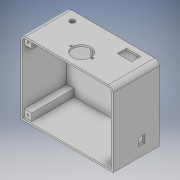
# Autodesk Inventor part: main_with_lid
Saved by Autodesk Inventor 2019 (Build 230136000, 136)
## iProperties
Created: 2019-03-27
Part Number: main_with_lid
Material: Generic
Document SubType Name: Modeling
Designer: hayes107
Density: 1 g/cm^3
Appearance: Default
Author: hayes107
Autodesk Inventor part; units mm, degrees
ref_plane "YZ Plane" through (0, 0, 0) normal (1, 0, 0) x (0, 1, 0)
ref_plane "XZ Plane" through (0, 0, 0) normal (0, 1, 0) x (-1, 0, 0)
ref_plane "XY Plane" through (0, 0, 0) normal (0, 0, 1) x (1, 0, 0)
sketch "Sketch1" plane through (0, 0, 0) normal (0, 0, 1) x (1, 0, 0)
  line L0 (0, 132.6086) -> (127, 132.6086)
  line L1 (127, 132.6086) -> (127, 31.0086)
  line L2 (127, 31.0086) -> (0, 31.0086)
  line L3 (0, 31.0086) -> (0, 132.6086)
  point P0 (0, 0)
  dimension "d0" = 101.6
  dimension "d1" = 127
  constraints: 8 end point, 2 parallel, 1 horizontal, 1 perpendicular
  measures "d0" distance between parallel lines of L2 L0
  measures "d1" distance between parallel lines of L1 L3
extrude "Extrusion1" add sketch "Sketch1" along normal blind 63.5
fillet "Fillet1" radius 6.35 1 edges at (127, 132.6086, 31.75)
fillet "Fillet2" radius 6.35 1 edges at (0, 132.6086, 31.75)
shell "Shell1" thickness 2.54 removed faces 1 at (82.55, 64.8753, 63.5)
sketch "Sketch16" plane through (0, 0, 0) normal (0, 0, -1) x (-1, 0, 0)
  line L0 (-91.3384, 109.6724) -> (-35.6616, 109.6724)
  line L1 (-35.6616, 109.6724) -> (-35.6616, 69.1086)
  line L2 (-35.6616, 69.1086) -> (-91.3384, 69.1086)
  line L3 (-91.3384, 69.1086) -> (-91.3384, 109.6724)
  line L4 (-127, 31.0086) -> (0, 31.0086) projected
  line L5 (0, 31.0086) -> (0, 126.2586) projected
  point P0 (0, 0)
  dimension "d69" = 40.5638
  dimension "d70" = 55.6768
  dimension "d71" = 38.1
  dimension "d72" = 35.6616
  constraints: 8 end point, 2 parallel, 1 horizontal, 1 perpendicular
  measures "d69" distance between parallel lines of L2 L0
  measures "d70" distance between parallel lines of L1 L3
  measures "d71" distance between parallel lines of L4 L2
  measures "d72" distance between parallel lines of L5 L1
extrude "Extrusion5" cut sketch "Sketch16" against normal blind 2.54
sketch "Sketch17" plane through (0, 0, 0) normal (0, 0, -1) x (-1, 0, 0)
  line L0 (-91.3384, 69.1086) -> (-91.3384, 109.6724) projected
  line L1 (-91.3384, 109.6724) -> (-35.6616, 109.6724) projected
  line L2 (-35.6616, 69.1086) -> (-91.3384, 69.1086) projected
  line L3 (-35.6616, 109.6724) -> (-35.6616, 69.1086) projected
  point P0 (0, 0)
  point P1 (-94.1832, 106.8276)
  point P2 (-94.1832, 71.9534)
  point P3 (-32.8168, 71.9534)
  point P4 (-32.8168, 106.8276)
  dimension "d75" = 2.8448
  dimension "d76" = 2.8448
  dimension "d77" = 2.8448
  dimension "d78" = 2.8448
  dimension "d305" = 2.8448
  dimension "d306" = 2.8448
  dimension "d307" = 2.8448
  measures "d75" distance from line of L0 point (-94.183, 106.828)
  measures "d76" distance from line of L1 point (-94.183, 106.828)
  measures "d77" distance from line of L2 point (-94.183, 71.953)
  measures "d78" distance from line of L3 point (-32.817, 71.953)
  measures "d305" distance from line of L2 point (-32.817, 71.953)
  measures "d306" distance from line of L3 point (-32.817, 106.828)
  measures "d307" distance from line of L1 point (-32.817, 106.828)
hole "Hole2" at (32.8168, 106.8276, 0) at (32.8168, 71.9534, 0) at (94.1832, 71.9534, 0) at (94.1832, 106.8276, 0) direction (0, 0, 1) diameter 2.6416 depth 12.7 tip angle 118
sketch "Sketch18" plane through (127, 31.0086, 63.5) normal (1, 0, 0) x (0, 0, -1)
  line L0 (35.052, 24.0792) -> (43.18, 24.0792)
  line L1 (43.18, 24.0792) -> (43.18, 13.6652)
  line L2 (43.18, 13.6652) -> (35.052, 13.6652)
  line L3 (35.052, 13.6652) -> (35.052, 24.0792)
  line L4 (63.5, 95.25) -> (63.5, 0) projected
  line L5 (63.5, 0) -> (0, 0) projected
  point P0 (63.5, -31.0086)
  dimension "d86" = 20.32
  dimension "d87" = 8.128
  dimension "d88" = 10.414
  dimension "d89" = 13.6652
  constraints: 8 end point, 2 parallel, 1 horizontal, 1 perpendicular
  measures "d86" distance between parallel lines of L4 L1
  measures "d87" distance between parallel lines of L3 L1
  measures "d88" distance between parallel lines of L2 L0
  measures "d89" distance between parallel lines of L2 L5
extrude "Extrusion6" cut sketch "Sketch18" against normal blind 2.54
sketch "Sketch26" plane through (120.65, 132.6086, 63.5) normal (0, 1, 0) x (1, 0, 0)
  line L0 (-107.95, 2.54) -> (-120.65, 2.54)
  line L1 (-120.65, 2.54) -> (-120.65, 63.5)
  line L2 (-120.65, 63.5) -> (-107.95, 63.5)
  line L3 (-107.95, 63.5) -> (-107.95, 2.54)
  line L4 (-120.65, 63.5) -> (-120.65, 0) projected
  line L5 (0, 0) -> (-114.3, 0) projected
  line L6 (-114.3, 63.5) -> (0, 63.5) projected
  line L7 (6.35, 31.75) -> (-6.35, 31.75)
  line L8 (-6.35, 31.75) -> (-6.35, 2.54)
  line L9 (-6.35, 2.54) -> (6.35, 2.54)
  line L10 (6.35, 2.54) -> (6.35, 31.75)
  line L11 (6.35, 0) -> (6.35, 63.5) projected
  dimension "d111" = 0
  dimension "d112" = 2.54
  dimension "d113" = 12.7
  dimension "d117" = 0
  dimension "d118" = 12.7
  dimension "d119" = 0
  dimension "d120" = 31.75
  dimension "d121" = 2.54
  constraints: 16 end point, 4 parallel, 2 horizontal, 2 perpendicular
  measures "d111" distance between parallel lines of L4 L1
  measures "d112" distance between parallel lines of L5 L0
  measures "d113" distance between parallel lines of L3 L1
  measures "d117" distance between parallel lines of L6 L2
  measures "d118" distance between parallel lines of L8 L10
  measures "d119" distance between parallel lines of L11 L10
  measures "d120" distance between parallel lines of L6 L7
  measures "d121" distance between parallel lines of L5 L9
sketch "Sketch27" plane through (0, 31.0086, 0) normal (0, -1, 0) x (1, 0, 0)
  line L0 (114.3, 60.96) -> (127, 60.96)
  line L1 (127, 60.96) -> (127, 31.75)
  line L2 (127, 31.75) -> (114.3, 31.75)
  line L3 (114.3, 31.75) -> (114.3, 60.96)
  line L4 (0, 63.5) -> (127, 63.5) projected
  line L5 (127, 0) -> (127, 63.5) projected
  line L6 (127, 0) -> (0, 0) projected
  line L7 (0, 60.96) -> (12.7, 60.96)
  line L8 (12.7, 60.96) -> (12.7, 0)
  line L9 (12.7, 0) -> (0, 0)
  line L10 (0, 0) -> (0, 60.96)
  line L11 (0, 0) -> (0, 63.5) projected
  dimension "d122" = 12.7
  dimension "d123" = 2.54
  dimension "d124" = 0
  dimension "d125" = 31.75
  dimension "d126" = 12.7
  dimension "d128" = 2.54
  dimension "d129" = 0
  dimension "d178" = 0
  constraints: 16 end point, 4 parallel, 2 horizontal, 2 perpendicular
  measures "d122" distance between parallel lines of L1 L3
  measures "d123" distance between parallel lines of L4 L0
  measures "d124" distance between parallel lines of L5 L1
  measures "d125" distance between parallel lines of L6 L2
  measures "d126" distance between parallel lines of L8 L10
  measures "d128" distance between parallel lines of L4 L7
  measures "d129" distance between parallel lines of L11 L10
  measures "d178" distance between parallel lines of L6 L9
sketch "Sketch30" plane through (120.65, 132.6086, 63.5) normal (0, 1, 0) x (1, 0, 0)
  circle A0 centre (-57.15, 20.32) radius 12.7
  line L0 (-120.65, 63.5) -> (-120.65, 0) projected
  line L1 (0, 0) -> (-114.3, 0) projected
  point P0 (-71.882, 20.32)
  point P1 (-42.418, 20.32)
  dimension "d189" = 63.5
  dimension "d190" = 20.32
  dimension "d191" = 25.4
  dimension "d192" = 14.732
  dimension "d193" = 14.732
  constraints: 1 centre point
  measures "d189" distance from line of L0 A0.centre
  measures "d190" distance from line of L1 A0.centre
  measures "d191" diameter of A0
  measures "d192" distance of point (-71.882, 20.32) A0.centre
  measures "d193" distance of A0.centre point (-42.418, 20.32)
hole "Hole5" at (78.232, 132.6086, 43.18) at (48.768, 132.6086, 43.18) direction (0, -1, 0) diameter 3.048 depth 12.7 tip angle 118
sketch "Sketch31" plane through (120.65, 132.6086, 63.5) normal (0, 1, 0) x (1, 0, 0)
  line L0 (0, 0) -> (-114.3, 0) projected
  line L1 (-120.65, 63.5) -> (-120.65, 0) projected
  point P0 (-57.15, 20.32)
  dimension "d201" = 20.32
  dimension "d202" = 63.5
  measures "d201" distance from line of L0 point (-57.15, 20.32)
  measures "d202" distance from line of L1 point (-57.15, 20.32)
hole "Hole6" at (63.5, 132.6086, 43.18) direction (0, -1, 0) diameter 25.4 depth 12.7 tip angle 118
sketch "Sketch32" plane through (120.65, 132.6086, 63.5) normal (0, 1, 0) x (1, 0, 0)
  line L0 (-30.988, 55.88) -> (-11.43, 55.88)
  line L1 (-11.43, 55.88) -> (-11.43, 43.18)
  line L2 (-11.43, 43.18) -> (-30.988, 43.18)
  line L3 (-30.988, 43.18) -> (-30.988, 55.88)
  line L4 (-114.3, 63.5) -> (0, 63.5) projected
  line L5 (6.35, 0) -> (6.35, 63.5) projected
  point P0 (-120.65, 63.5)
  dimension "d210" = 19.558
  dimension "d211" = 12.7
  dimension "d212" = 7.62
  dimension "d213" = 17.78
  constraints: 8 end point, 2 parallel, 1 horizontal, 1 perpendicular
  measures "d210" distance between parallel lines of L1 L3
  measures "d211" distance between parallel lines of L2 L0
  measures "d212" distance between parallel lines of L4 L0
  measures "d213" distance between parallel lines of L5 L1
extrude "Extrusion11" cut sketch "Sketch32" against normal blind 25.4
sketch "Sketch33" plane through (120.65, 132.6086, 63.5) normal (0, 1, 0) x (1, 0, 0)
  circle A0 centre (-100.33, 50.8) radius 3.556
  line L0 (-114.3, 63.5) -> (0, 63.5) projected
  line L1 (-120.65, 63.5) -> (-120.65, 0) projected
  dimension "d216" = 12.7
  dimension "d217" = 20.32
  dimension "d218" = 7.112
  constraints: 1 centre point
  measures "d216" distance from line of L0 A0.centre
  measures "d217" distance from line of L1 A0.centre
  measures "d218" diameter of A0
hole "Hole7" at (20.32, 132.6086, 12.7) direction (0, -1, 0) diameter 7.112 depth 12.7 tip angle 118
extrude "Extrusion12" add sketch "Sketch27" against normal blind 12.7 contours L6 L10 L7 L8
extrude "Extrusion13" add sketch "Sketch26" against normal blind 12.7 contours L0 L1 L2 L3
fillet "Fillet4" radius 6.35 1 edges at (0, 132.6086, 30.48)
sketch "Sketch37" plane through (2.54, 119.9086, 60.96) normal (0, 0, 1) x (1, 0, 0)
  line L0 (10.16, 10.16) -> (10.16, 0) projected
  line L1 (10.16, 0) -> (0, 0) projected
  line L2 (0, -76.2) -> (10.16, -76.2) projected
  line L3 (10.16, -86.36) -> (10.16, -76.2) projected
  point P0 (-2.54, -119.9086)
  point P1 (5.08, 5.08)
  point P2 (5.08, -81.28)
  dimension "d265" = 5.08
  dimension "d266" = 5.08
  dimension "d267" = 5.08
  dimension "d268" = 5.08
  measures "d265" distance from line of L0 point (5.08, 5.08)
  measures "d266" distance from line of L1 point (5.08, 5.08)
  measures "d267" distance from line of L2 point (5.08, -81.28)
  measures "d268" distance from line of L3 point (5.08, -81.28)
hole "Hole9" at (7.62, 124.9886, 60.96) at (7.62, 38.6286, 60.96) direction (0, 0, -1) diameter 2.6416 depth 12.7 tip angle 118
thread "Thread17" size "1/16" designation "1/16 - 27 NPT" standard "NPT for PVC Pipe and Fitting" full length
thread "Thread18" size "1/16" designation "1/16 - 27 NPT" standard "NPT for PVC Pipe and Fitting" full length
sketch "Sketch38" plane through (124.46, 33.5486, 2.54) normal (-1, 0, 0) x (0, 0, 1)
  line L0 (58.42, 59.69) -> (59.69, 59.69)
  line L1 (59.69, 59.69) -> (59.69, 34.29)
  line L2 (59.69, 34.29) -> (58.42, 34.29)
  line L3 (58.42, 34.29) -> (58.42, 59.69)
  line L4 (60.96, 92.71) -> (60.96, 0) projected
  line L5 (60.96, 92.71) -> (0, 92.71) projected
  line L6 (0, 0) -> (60.96, 0) projected
  point P0 (-2.54, -33.5486)
  dimension "d280" = 25.4
  dimension "d281" = 1.27
  dimension "d282" = 1.27
  dimension "d308" = 34.29
  constraints: 8 end point, 2 parallel, 1 horizontal, 1 perpendicular
  measures "d280" distance between parallel lines of L2 L0
  measures "d281" distance between parallel lines of L3 L1
  measures "d282" distance between parallel lines of L1 L4
  measures "d308" distance from line of L6 L1.end
extrude "Extrusion14" cut sketch "Sketch38" against normal blind 1.27
body "Solid1"
